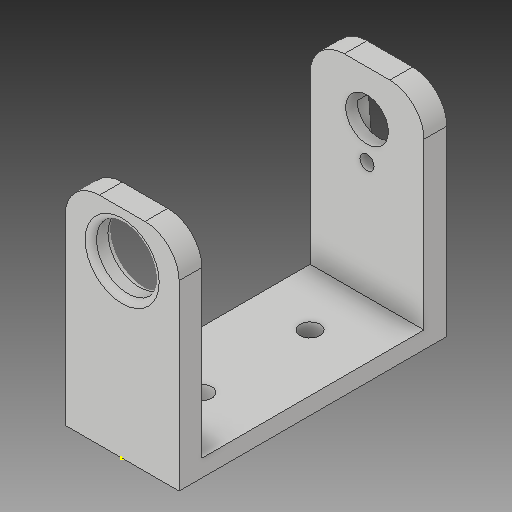
# Autodesk Inventor part: new_femur
Saved by Autodesk Inventor 2019 (Build 230136000, 136)
## iProperties
Created: 2019-02-03
Part Number: new_femur
Material: Generic
Document SubType Name: Modeling
Designer: Daniel
Density: 1 g/cm^3
Appearance: Default
Author: Daniel
Autodesk Inventor part; units mm, degrees
note: some values were not read from the file. Chosen so that the rebuilt part matches the saved one: direction of "Hole1"; direction of "Hole4"; direction of "Hole5".
ref_plane "YZ Plane" through (0, 0, 0) normal (1, 0, 0) x (0, 1, 0)
ref_plane "XZ Plane" through (0, 0, 0) normal (0, 1, 0) x (-1, 0, 0)
ref_plane "XY Plane" through (0, 0, 0) normal (0, 0, 1) x (1, 0, 0)
sketch "Sketch1" plane through (0, 0, 0) normal (0, 1, 0) x (-1, 0, 0)
  line L0 (14, 0) -> (-14, 0) projected
  line L1 (0, -32.9) -> (0, 32.9) projected
  line L2 (10, 23.5) -> (-10, 23.5)
  line L3 (-10, 23.5) -> (-10, -23.5)
  line L4 (-10, -23.5) -> (10, -23.5)
  line L5 (10, -23.5) -> (10, 23.5)
  point P0 (0, 0)
  dimension "d0" = 47
  dimension "d1" = 20
  constraints: 8 end point, 2 parallel, 1 horizontal, 1 perpendicular, 2 other
  measures "d0" distance between parallel lines of L4 L2
  measures "d1" distance between parallel lines of L3 L5
extrude "Extrusion1" add sketch "Sketch1" along normal blind 3
sketch "Sketch2" plane through (0, 3, 0) normal (0, 1, 0) x (1, 0, 0)
  line L0 (-10, -23.5) -> (10, -23.5) projected
  line L1 (10, -23.5) -> (10, 23.5) projected
  line L2 (10, 23.5) -> (-10, 23.5) projected
  line L3 (-10, 23.5) -> (-10, -23.5) projected
  line L4 (-10, -23.5) -> (10, -23.5)
  line L5 (10, -23.5) -> (10, -19.5)
  line L6 (10, -19.5) -> (-10, -19.5)
  line L7 (-10, -19.5) -> (-10, -23.5)
  line L8 (-10, 19.5) -> (10, 19.5)
  line L9 (10, 19.5) -> (10, 23.5)
  line L10 (10, 23.5) -> (-10, 23.5)
  line L11 (-10, 23.5) -> (-10, 19.5)
  line L12 (-10, -23.5) -> (10, -23.5) projected
  line L13 (-10, 23.5) -> (-10, -23.5) projected
  line L14 (10, -23.5) -> (10, 23.5) projected
  line L15 (10, 23.5) -> (-10, 23.5) projected
  point P0 (0, 0)
  dimension "d4" = 4
  dimension "d5" = 4
  constraints: 16 end point, 4 collinear, 4 parallel, 2 horizontal, 2 perpendicular, 2 point on line
  measures "d4" distance between parallel lines of L0 L6
  measures "d5" distance between parallel lines of L2 L8
extrude "Extrusion2" add sketch "Sketch2" along normal blind 35 contours L3 L6 L1 L0 | L3 L2 L1 L8
sketch "Sketch3" plane through (-10, 0, 23.5) normal (0, 0, 1) x (1, 0, 0)
  point P0 (10, 0)
sketch "Sketch4" plane through (-10, 0, 23.5) normal (0, 0, 1) x (1, 0, 0)
  line L0 (0, 0) -> (20, 0) projected
  line L1 (20, 0) -> (20, 38) projected
  line L2 (0, 38) -> (20, 38) projected
  line L3 (0, 0) -> (0, 38) projected
  point P0 (10, 0)
  point P1 (10, 30)
  dimension "d8" = 10
  dimension "d9" = 8
  measures "d8" distance from line of L3 point (10, 30)
  measures "d9" distance from line of L2 point (10, 30)
hole "Hole1" at (0, 30, 23.5) direction (0, 0, -1) diameter 11 depth 43
fillet "Fillet1" radius 6 4 edges at (10, 38, -21.5) (-10, 38, -21.5) (10, 38, 21.5) (-10, 38, 21.5)
sketch "Sketch8" plane through (0, 0, 0) normal (0, -1, 0) x (1, 0, 0)
  line L0 (-10, 23.5) -> (10, 23.5) projected
  line L1 (-10, -23.5) -> (-10, 23.5) projected
  line L2 (10, -23.5) -> (-10, -23.5) projected
  line L3 (10, 23.5) -> (10, -23.5) projected
  line L4 (-14, 0) -> (14, 0) projected
  line L5 (0, -32.9) -> (0, 32.9) projected
  line L6 (10, -19.5) -> (-10, -19.5) projected
  line L7 (-10, 19.5) -> (10, 19.5) projected
  point P0 (0, 0)
  point P1 (0, -9.5)
  point P2 (0, 9.5)
  dimension "d37" = 10
  dimension "d38" = 10
  dimension "d75" = 19
  constraints: 2 point on line
  measures "d37" distance from line of L6 point (0, -9.5)
  measures "d38" distance from line of L7 point (0, 9.5)
  measures "d75" distance of point (0, 9.5) point (0, -9.5)
hole "Hole3" at (0, 0, 9.5) at (0, 0, -9.5) direction (0, 1, 0) diameter 3.5 end through all
sketch "Sketch10" plane through (10, 0, -23.5) normal (0, 0, -1) x (-1, 0, 0)
  arc A0 (20, 32) -> (14, 38) centre (14, 32) ccw projected
  line L0 (6, 38) -> (14, 38) projected
  arc A1 (6, 38) -> (0, 32) centre (6, 32) ccw projected
  line L1 (0, 0) -> (0, 32) projected
  line L2 (0, 0) -> (20, 0) projected
  line L3 (20, 0) -> (20, 32) projected
  circle A2 centre (10, 30) radius 5.5 projected
  circle A3 centre (10, 30) radius 3.75
  circle A4 centre (10, 16) radius 2.5
  line L4 (-6.7241, 13.5) -> (37.2046, 13.5) construction
  line L5 (6.25, 30) -> (7.5505, 15.5)
  line L6 (13.75, 30) -> (12.4495, 15.5)
  point P0 (10, 0)
  dimension "d47" = 16.5
  dimension "d48" = 7.5
  dimension "d49" = 5
  dimension "d50" = 10
  dimension "d51" = 2
  dimension "d52" = 2
  dimension "d53" = 8
  dimension "d54" = 8
  constraints: 6 end point, 4 point on circle, 2 centre point, 1 coincident, 1 horizontal, 1 tangent
  measures "d47" distance from line of L4 A3.centre
  measures "d48" diameter of A3
  measures "d49" diameter of A4
  measures "d50" distance from line of L1 A4.centre
  measures "d51" distance from line of L4 L6.end
  measures "d52" distance from line of L4 L5.end
  measures "d53" distance from line of L0 L6.start
  measures "d54" distance from line of L0 L5.start
extrude "Extrusion4" cut sketch "Sketch10" against normal blind 2 contours L5 A3 L6 A2 | A2 L6 A4 L5 | L5 A3 L6 | A4 L6 L5 picked at (9.6017, 25.1271)
sketch "Sketch11" plane through (10, 0, -21.5) normal (0, 0, -1) x (-1, 0, 0)
  line L0 (7.5505, 15.5) -> (6.25, 30) projected
  arc A0 (7.5505, 15.5) -> (12.4495, 15.5) centre (10, 16) ccw projected
  line L1 (13.75, 30) -> (12.4495, 15.5) projected
  arc A1 (13.75, 30) -> (6.25, 30) centre (10, 30) ccw projected
  point P0 (10, 0)
  constraints: 1 coincident
hole "Hole4" at (0, 30, -21.5) direction (0, 0, 1) diameter 7.5 depth 41
sketch "Sketch12" plane through (10, 0, -21.5) normal (0, 0, -1) x (-1, 0, 0)
  arc A0 (6.3099, 29.3327) -> (13.6901, 29.3327) centre (10, 30) ccw projected
  line L0 (7.5505, 15.5) -> (6.3099, 29.3327) projected
  arc A1 (7.5505, 15.5) -> (12.4495, 15.5) centre (10, 16) ccw projected
  line L1 (13.6901, 29.3327) -> (12.4495, 15.5) projected
  line L2 (0, 0) -> (0, 32) projected
  point P0 (10, 0)
  point P1 (10, 23.5)
  dimension "d64" = 6.5
  dimension "d65" = 10
  measures "d64" distance of A0.centre point (10, 23.5)
  measures "d65" distance from line of L2 point (10, 23.5)
hole "Hole5" at (0, 23.5, -21.5) direction (0, 0, 1) diameter 2.5 depth 41
fillet "Fillet2" radius 1 1 edges at (0, 35.5, 19.5)
fillet "Fillet3" radius 1 1 edges at (0, 35.5, 23.5)
body "Solid1"
